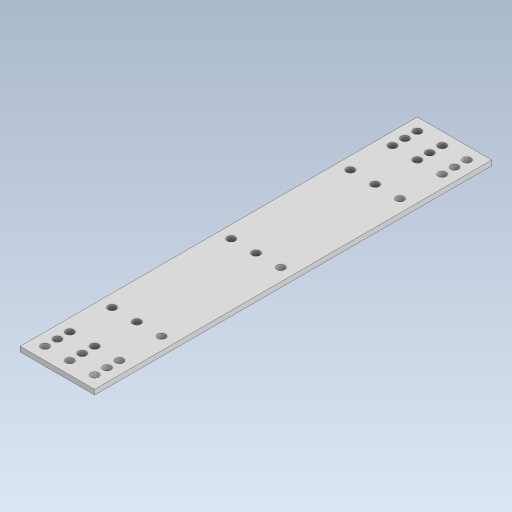
# Autodesk Inventor part: Fix Bracker Holder Gripper
Saved by Autodesk Inventor 2023.5 (Build 275446000, 446)
## iProperties
Created: 2025-10-01
Part Number: Fix Bracker Holder Gripper
Material: Generic
Document SubType Name: Modeling
Designer: Guntur
Density: 1 g/cm^3
Appearance: Default
Author: Guntur
## iProperties of the stored document Fix Bracker Holder Gripper_3DPrint.ipt
Created: 2025-10-12
Part Number: Fix Bracker Holder Gripper_3DPrint
Material: Generic
Document SubType Name: Modeling
Designer: Guntur
Density: 1 g/cm^3
Appearance: Default
Author: Guntur
Autodesk Inventor part; units mm, degrees
ref_plane "YZ Plane" through (0, 0, 0) normal (1, 0, 0) x (0, 1, 0)
ref_plane "XZ Plane" through (0, 0, 0) normal (0, 1, 0) x (-1, 0, 0)
ref_plane "XY Plane" through (0, 0, 0) normal (0, 0, 1) x (1, 0, 0)
sketch "Sketch1" plane through (0, 0, 0) normal (0, 1, 0) x (-1, 0, 0)
  line L0 (88, 0) -> (-78, 0) construction
  line L1 (0, 88) -> (0, -110) construction
  line L2 (0, 0) -> (30, 0)
  line L3 (30, 0) -> (30, -80)
  line L4 (30, -80) -> (0, -80)
  line L5 (0, -80) -> (0, 0)
  circle A0 centre (25, -75) radius 1.6
  circle A1 centre (5, -75) radius 1.6
  circle A2 centre (15, -75) radius 1.6
  circle A3 centre (25, -70) radius 1.6
  circle A4 centre (15, -70) radius 1.6
  circle A5 centre (5, -70) radius 1.6
  circle A6 centre (25, -65) radius 1.6
  circle A7 centre (15, -65) radius 1.6
  circle A8 centre (5, -65) radius 1.6
  line L6 (30, 0) -> (30, 80)
  line L7 (30, 80) -> (0, 80)
  circle A9 centre (25, 75) radius 1.6
  circle A10 centre (5, 75) radius 1.6
  circle A11 centre (15, 75) radius 1.6
  circle A12 centre (25, 70) radius 1.6
  circle A13 centre (15, 70) radius 1.6
  circle A14 centre (5, 70) radius 1.6
  circle A15 centre (25, 65) radius 1.6
  circle A16 centre (15, 65) radius 1.6
  circle A17 centre (5, 65) radius 1.6
  circle A18 centre (25, 0) radius 1.6
  circle A19 centre (5, 0) radius 1.6
  circle A20 centre (15, 0) radius 1.6
  line L8 (0, 80) -> (0, 0)
  circle A21 centre (25, -48) radius 1.6
  circle A22 centre (15, -48) radius 1.6
  circle A23 centre (5, -48) radius 1.6
  circle A24 centre (25, 48) radius 1.6
  circle A25 centre (15, 48) radius 1.6
  circle A26 centre (5, 48) radius 1.6
  dimension "d0" = 30
  dimension "d1" = 80
  dimension "d2" = 3.2
  dimension "d3" = 5
  dimension "d4" = 5
  dimension "d5" = 3.2
  dimension "d6" = 3.2
  dimension "d7" = 3.2
  dimension "d8" = 5
  dimension "d9" = 3.2
  dimension "d10" = 3.2
  dimension "d11" = 3.2
  dimension "d12" = 5
  dimension "d13" = 3.2
  dimension "d14" = 3.2
  dimension "d15" = 3.2
  dimension "d17" = 3.2
  dimension "d18" = 3.2
  dimension "d21" = 3.2
  dimension "d22" = 48
  dimension "d23" = 3.2
  dimension "d24" = 3.2
  constraints: 27 centre point, 18 end point, 14 symmetric about line, 3 horizontal, 2 parallel, 2 point on line, 2 vertical, 1 collinear, 1 midpoint, 1 perpendicular, 13 other
  measures "d0" distance of L3.end L4.end
  measures "d1" distance of L2.end L3.end
  measures "d2" diameter of A0
  measures "d3" distance from line of L3 A0.centre
  measures "d4" distance from line of L4 A0.centre
  measures "d5" diameter of A1
  measures "d6" diameter of A2
  measures "d7" diameter of A3
  measures "d8" distance of A0.centre A3.centre
  measures "d9" diameter of A4
  measures "d10" diameter of A5
  measures "d11" diameter of A6
  measures "d12" distance of A3.centre A6.centre
  measures "d13" diameter of A7
  measures "d14" diameter of A8
  measures "d15" diameter of A18
  measures "d17" diameter of A19
  measures "d18" diameter of A20
  measures "d21" diameter of A21
  measures "d22" distance of A21.centre A18.centre
  measures "d23" diameter of A22
  measures "d24" diameter of A23
extrude "Extrusion1" add sketch "Sketch1" along normal blind 2 contours A18 L2 A20 A19 L8 L7 L6 | L2 L3 L4 L5 A19 A20 A18
body "Solid1"
